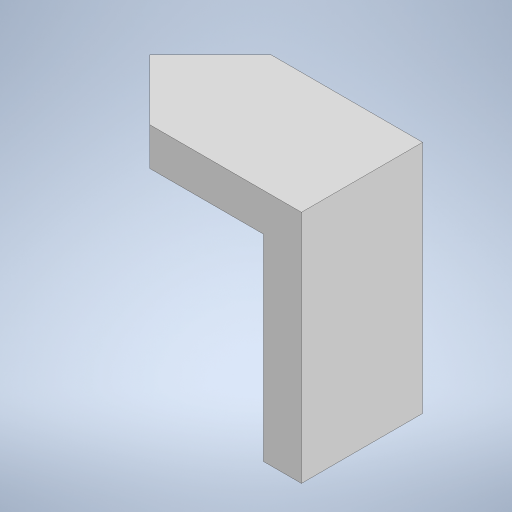
# Autodesk Inventor part: Connecting pt.1
Saved by Autodesk Inventor 2023 (Build 270158000, 158)
## iProperties
Created: 2025-04-14
Part Number: Connecting pt.1
Material: Generic
Document SubType Name: Modeling
Designer: 1khanhan2
Density: 1 g/cm^3
Appearance: Default
Author: 1khanhan2
Autodesk Inventor part; units mm, degrees
ref_plane "YZ Plane" through (0, 0, 0) normal (1, 0, 0) x (0, 1, 0)
ref_plane "XZ Plane" through (0, 0, 0) normal (0, 1, 0) x (-1, 0, 0)
ref_plane "XY Plane" through (0, 0, 0) normal (0, 0, 1) x (1, 0, 0)
sketch "Sketch1" plane through (0, 0, 0) normal (0, 1, 0) x (-1, 0, 0)
  line L0 (0, 0) -> (0, -16)
  line L1 (8, -8) -> (0, 0)
  line L2 (8, -8) -> (0, -16)
  line L3 (0, 0) -> (-20, 0)
  line L4 (-20, 0) -> (-20, -16)
  line L5 (-20, -16) -> (0, -16)
  dimension "d0" = 16
  dimension "d2" = 20
  constraints: 12 end point, 2 perpendicular, 1 horizontal, 1 vertical
  measures "d0" distance of L0.start L0.end
  measures "d2" distance of L0.start L3.end
extrude "Extrusion1" add sketch "Sketch1" along normal blind 5
sketch "Sketch2" plane through (0, 0, 0) normal (0, -1, 0) x (1, 0, 0)
  line L0 (20, -16) -> (0, -16) projected
  line L1 (20, -16) -> (15, -16)
  line L2 (15, -16) -> (15, 0)
  line L3 (0, 0) -> (20, 0) projected
  line L4 (20, 0) -> (20, -16) projected
  line L5 (20, 0) -> (20, -16)
  line L6 (20, -16) -> (18.5, -16)
  line L7 (15, -16) -> (15, -14.5)
  line L8 (15, -16) -> (16.5, -16)
  line L9 (16.5, -14.5) -> (18.5, -14.5)
  line L10 (18.5, -14.5) -> (18.5, -1.5)
  line L11 (18.5, -1.5) -> (16.5, -1.5)
  line L12 (16.5, -1.5) -> (16.5, -14.5)
  dimension "d5" = 5
  dimension "d8" = 1.5
  dimension "d9" = 1.5
  dimension "d11" = 13
  constraints: 20 end point, 5 point on line, 3 perpendicular, 1 collinear, 1 vertical
  measures "d5" distance of L0.start L1.end
  measures "d8" distance of L0.start L6.end
  measures "d9" distance of L6.end L9.end
  measures "d11" distance of L9.end L10.end
extrude "Extrusion2" add sketch "Sketch2" along normal blind 26
extrude "Extrusion3" add sketch "Sketch2" along normal blind 27 contours L12 L11 L10 L9
body "Solid1"
